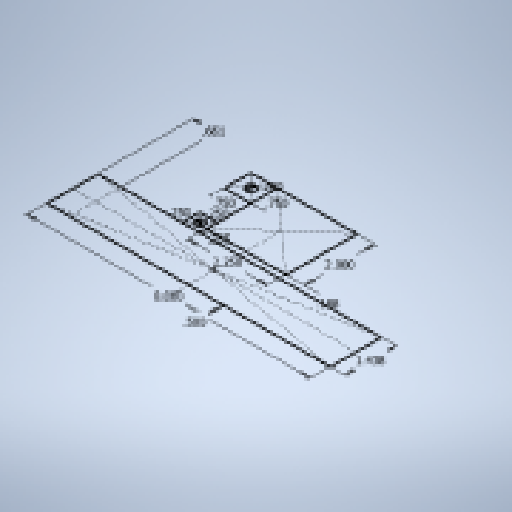
# Autodesk Inventor part: Chassis
Saved by Autodesk Inventor 2023.1 (Build 271208000, 208)
## iProperties
Created: 2022-12-23
Part Number: Chassis
Material: UHMW, White
Document SubType Name: Modeling
Designer: Nathan Cai
Density: 0.94 g/cm^3
Appearance: Smooth - White
Author: Nathan Cai
Autodesk Inventor part; units mm, degrees
ref_plane "YZ Plane" through (0, 0, 0) normal (1, 0, 0) x (0, 1, 0)
ref_plane "XZ Plane" through (0, 0, 0) normal (0, 1, 0) x (-1, 0, 0)
ref_plane "XY Plane" through (0, 0, 0) normal (0, 0, 1) x (1, 0, 0)
sketch "Sketch1" plane through (0, 0, 0) normal (0, 1, 0) x (-1, 0, 0)
  line L0 (28.575, -103.1875) -> (-28.575, -103.1875) construction
  line L1 (-28.575, -103.1875) -> (-28.575, -52.3875)
  line L2 (-28.575, -52.3875) -> (28.575, -52.3875)
  line L3 (28.575, -52.3875) -> (28.575, -103.1875)
  line L4 (28.575, -103.1875) -> (-28.575, -52.3875) construction
  line L5 (-28.575, -103.1875) -> (28.575, -52.3875) construction
  line L6 (0, -77.7875) -> (0, 0) construction
  line L7 (47.625, -103.1875) -> (28.575, -103.1875)
  line L8 (28.575, -103.1875) -> (28.575, -84.1375)
  line L9 (28.575, -84.1375) -> (47.625, -84.1375) construction
  line L10 (47.625, -84.1375) -> (47.625, -103.1875) construction
  line L11 (47.625, -103.1875) -> (28.575, -84.1375) construction
  line L12 (28.575, -103.1875) -> (47.625, -84.1375) construction
  circle A0 centre (38.1, -93.6625) radius 3.556
  line L13 (101.6, -49.2125) -> (-101.6, -49.2125)
  line L14 (-101.6, -49.2125) -> (-101.6, -12.7)
  line L15 (-101.6, -12.7) -> (101.6, -12.7)
  line L16 (101.6, -12.7) -> (101.6, -49.2125)
  line L17 (101.6, -49.2125) -> (-101.6, -12.7) construction
  line L18 (-101.6, -49.2125) -> (101.6, -12.7) construction
  line L19 (84.8, -49.2125) -> (84.8, -12.7) construction
  line L20 (-101.6, -30.9563) -> (101.6, -30.9563) construction
  circle A1 centre (34.925, -55.5625) radius 3.3655
  line L21 (41.275, -61.9125) -> (28.575, -61.9125)
  line L22 (28.575, -61.9125) -> (28.575, -49.2125)
  line L23 (28.575, -49.2125) -> (41.275, -49.2125)
  line L24 (41.275, -49.2125) -> (41.275, -61.9125)
  line L25 (41.275, -61.9125) -> (28.575, -49.2125) construction
  line L26 (28.575, -61.9125) -> (41.275, -49.2125) construction
  line L27 (34.925, -55.5625) -> (34.925, -7.9375) construction
  line L28 (41.275, -12.7) -> (28.575, -12.7)
  line L29 (28.575, -12.7) -> (28.575, -3.175) construction
  line L30 (28.575, -3.175) -> (41.275, -3.175)
  line L31 (41.275, -3.175) -> (41.275, -12.7)
  line L32 (41.275, -12.7) -> (28.575, -3.175) construction
  line L33 (28.575, -12.7) -> (41.275, -3.175) construction
  circle A2 centre (34.925, -7.9375) radius 3.3655
  circle A3 centre (38.1, -93.6625) radius 9.525
  line L34 (101.6, -49.2125) -> (60.325, -49.2125)
  line L35 (60.325, -49.2125) -> (60.325, -68.2625) construction
  line L36 (60.325, -68.2625) -> (101.6, -68.2625)
  line L37 (101.6, -68.2625) -> (101.6, -49.2125)
  line L38 (41.275, -52.3875) -> (60.325, -52.3875)
  line L39 (101.6, -7.9375) -> (41.275, -7.9375) construction
  line L40 (101.6, -7.9375) -> (101.6, -12.7)
  line L41 (101.6, -7.9375) -> (41.275, -3.175)
  line L42 (92.075, -49.2125) -> (92.075, -12.7)
  line L43 (60.325, -68.2625) -> (46.747, -97.6568)
  line L44 (34.925, -61.9125) -> (34.925, -84.6822)
  line L45 (57.166, -52.3875) -> (42.0943, -85.0155)
  line L46 (28.575, -3.175) -> (0, -3.175)
  circle A4 centre (60.325, -61.9125) radius 1.1906
  line L47 (101.6, -61.9125) -> (84.8, -61.9125)
  line L48 (84.8, -61.9125) -> (84.8, -36.5125)
  line L49 (84.8, -36.5125) -> (101.6, -36.5125)
  line L50 (101.6, -36.5125) -> (101.6, -61.9125)
  line L51 (84.8, -49.2125) -> (101.6, -49.2125) construction
  line L52 (84.8, -61.9125) -> (65.75, -61.9125)
  line L53 (65.75, -61.9125) -> (65.75, -36.5125)
  line L54 (65.75, -36.5125) -> (84.8, -36.5125)
  line L55 (84.8, -36.5125) -> (84.8, -61.9125)
  circle A5 centre (60.325, -36.5125) radius 1.1906
  line L56 (96.8375, -36.5125) -> (96.8375, -12.7) construction
  circle A6 centre (96.8375, -33.3375) radius 1.1906
  circle A7 centre (96.8375, -12.7) radius 1.1906
  circle A8 centre (60.325, -36.5125) radius 3.175
  line L57 (60.325, -33.3375) -> (92.075, -33.3375)
  line L58 (57.166, -36.1945) -> (57.166, -52.3875)
  line L59 (-47.625, -103.1875) -> (-28.575, -103.1875)
  circle A9 centre (-38.1, -93.6625) radius 3.556
  circle A10 centre (-34.925, -55.5625) radius 3.3655
  line L60 (-41.275, -61.9125) -> (-28.575, -61.9125)
  line L61 (-41.275, -49.2125) -> (-41.275, -61.9125)
  line L62 (-28.575, -3.175) -> (-41.275, -3.175)
  circle A11 centre (-34.925, -7.9375) radius 3.3655
  circle A12 centre (-38.1, -93.6625) radius 9.525
  line L63 (-60.325, -68.2625) -> (-101.6, -68.2625)
  line L64 (-101.6, -68.2625) -> (-101.6, -49.2125)
  line L65 (-41.275, -52.3875) -> (-60.325, -52.3875)
  line L66 (-101.6, -7.9375) -> (-41.275, -3.175)
  line L67 (-92.075, -49.2125) -> (-92.075, -12.7)
  line L68 (-60.325, -68.2625) -> (-46.747, -97.6568)
  line L69 (-34.925, -61.9125) -> (-34.925, -84.6822)
  line L70 (-57.166, -52.3875) -> (-42.0943, -85.0155)
  line L71 (-28.575, -3.175) -> (0, -3.175)
  circle A13 centre (-60.325, -61.9125) radius 1.1906
  line L72 (-101.6, -61.9125) -> (-84.8, -61.9125)
  line L73 (-84.8, -61.9125) -> (-84.8, -36.5125)
  line L74 (-84.8, -36.5125) -> (-101.6, -36.5125)
  line L75 (-84.8, -61.9125) -> (-65.75, -61.9125)
  line L76 (-65.75, -61.9125) -> (-65.75, -36.5125)
  line L77 (-65.75, -36.5125) -> (-84.8, -36.5125)
  circle A14 centre (-60.325, -36.5125) radius 1.1906
  circle A15 centre (-96.8375, -33.3375) radius 1.1906
  circle A16 centre (-96.8375, -12.7) radius 1.1906
  circle A17 centre (-60.325, -36.5125) radius 3.175
  line L78 (-60.325, -33.3375) -> (-92.075, -33.3375)
  line L79 (-57.166, -36.1945) -> (-57.166, -52.3875)
  line L80 (-101.6, -7.9375) -> (-101.6, -12.7)
  line L81 (41.275, -61.9125) -> (62.6618, -38.662)
  line L82 (-41.275, -61.9125) -> (-62.6618, -38.662)
  circle A18 centre (96.8375, -65.0875) radius 1.1906
  circle A19 centre (96.8375, -65.0875) radius 3.175 construction
  line L83 (87.975, -63.5) -> (84.8, -63.5)
  line L84 (84.8, -63.5) -> (84.8, -34.925)
  line L85 (84.8, -34.925) -> (87.975, -34.925)
  line L86 (87.975, -34.925) -> (87.975, -63.5)
  line L87 (87.975, -63.5) -> (84.8, -34.925) construction
  line L88 (84.8, -63.5) -> (87.975, -34.925) construction
  line L89 (-84.8, -61.9125) -> (-84.8, -36.5125)
  line L90 (-84.8, -36.5125) -> (-84.8, -61.9125)
  circle A20 centre (-96.8375, -65.0875) radius 1.1906
  circle A21 centre (-96.8375, -65.0875) radius 3.175
  line L91 (-87.975, -63.5) -> (-84.8, -63.5)
  line L92 (-84.8, -63.5) -> (-84.8, -34.925)
  line L93 (-84.8, -34.925) -> (-87.975, -34.925)
  line L94 (-87.975, -34.925) -> (-87.975, -63.5)
  line L95 (-87.975, -63.5) -> (-84.8, -34.925) construction
  line L96 (-84.8, -63.5) -> (-87.975, -34.925) construction
  point P0 (0, -30.9563)
  point P1 (-57.166, -49.2125)
  point P2 (-92.075, -12.7)
  point P3 (57.166, -49.2125)
  point P4 (38.1, -103.1875)
  point P5 (-38.1, -103.1875)
  point P6 (-50.0365, -52.3875)
  point P7 (50.0365, -52.3875)
  point P8 (86.3875, -49.2125)
  point P9 (-84.8, -49.2125)
  point P10 (-84.8, -49.2125)
  point P11 (-86.3875, -49.2125)
  dimension "d0" = 57.15
  dimension "d1" = 50.8
  dimension "d2" = 19.05
  dimension "d3" = 19.05
  dimension "d4" = 7.112
  dimension "d7" = 203.2
  dimension "d8" = 36.5125
  dimension "d9" = 3.175
  dimension "d10" = 16.8
  dimension "d11" = 6.731
  dimension "d12" = 6.35
  dimension "d13" = 6.35
  dimension "d14" = 12.7
  dimension "d15" = 12.7
  dimension "d16" = 9.525
  dimension "d17" = 6.731
  dimension "d18" = 41.275
  dimension "d19" = 19.05
  dimension "d20" = 3.175
  dimension "d21" = 9.525
  dimension "d23" = 9.525
  dimension "d24" = 2.3813
  dimension "d25" = 6.35
  dimension "d26" = 16.8
  dimension "d27" = 25.4
  dimension "d29" = 19.05
  dimension "d32" = 25.4
  dimension "d37" = 4.7625
  dimension "d38" = 2.3813
  dimension "d39" = 2.3813
  dimension "d40" = 6.35
  dimension "d41" = 3.175
  dimension "d51" = 6.35
  dimension "d52" = 3.175
  dimension "d53" = 28.575
  dimension "d54" = 6.35
  constraints: 194 end point, 52 symmetric about line, 31 point on line, 22 centre point, 20 parallel, 18 midpoint, 17 perpendicular, 11 point on circle, 9 horizontal, 7 coincident, 4 tangent, 3 vertical, 1 concentric, 14 other
  measures "d0" distance of L1.end L2.end
  measures "d1" distance of L0.end L1.end
  measures "d2" distance of L8.end L9.end
  measures "d3" distance of L7.end L8.end
  measures "d4" diameter of A0
  measures "d7" distance of L14.end L15.end
  measures "d8" distance of L13.end L14.end
  measures "d9" distance between parallel lines of L13 L2
  measures "d10" distance between parallel lines of L16 L19
  measures "d11" diameter of A1
  measures "d12" distance from line of L3 L27.start
  measures "d13" distance from line of L13 L27.start
  measures "d14" distance from line of L6.end L15
  measures "d15" distance of L29.end L30.end
  measures "d16" distance of L28.end L29.end
  measures "d17" diameter of A2
  measures "d18" distance of L36.end L35.end
  measures "d19" distance of L35.end L34.end
  measures "d20" distance between parallel lines of L13 L38
  measures "d21" distance between parallel lines of L16 L42
  measures "d23" distance between parallel lines of L43 L45
  measures "d24" diameter of A4
  measures "d25" distance from line of L36 A4.centre
  measures "d26" distance of L48.end L49.end
  measures "d27" distance of L47.end L48.end
  measures "d29" distance of L53.end L54.end
  measures "d32" distance of A4.centre A5.centre
  measures "d37" distance between parallel lines of L16 L56
  measures "d38" diameter of A6
  measures "d39" diameter of A7
  measures "d40" diameter of A8
  measures "d41" distance from line of L49 A6.centre
  measures "d51" diameter of A19
  measures "d52" distance of L84.end L85.end
  measures "d53" distance of L83.end L84.end
  measures "d54" distance between parallel lines of L36 L52
extrude "Extrusion1" add sketch "Sketch1" along normal blind 25.4 contours L59 A12 L1 | A12 L69 L60 L1 | A12 | L60 L61 L13 L22 L2 L1 | L68 L63 A21 L72 L94 L91 L92 L75 L76 L13 L79 L70 A12 | L22 L13 L24 L21 L3 | L82 L65 L61 | L79 L13 L82 L65 | L63 L64 L72 A21 | A21 | L21 L44 A3 L3 | L65 L82 L13 L61 | L13 L76 L77 L92 L93 L94 L74 L67 L78 A17 L82 L79 | L72 L64 L13 L94 | L13 L81 L38 L24 | L82 A17 L79 | A3 L7 L3 | A3 | L24 L38 L81 | L13 L58 L38 L81 | A17 L79 | L14 L74 L67 L13 | L13 L67 L74 L94 | L45 L58 L13 L53 L52 L84 L83 L86 L47 L37 L36 L43 A3 | L58 L81 A8 L57 L42 L49 L86 L85 L84 L54 L53 L13 | L58 A8 L81 | L14 L15 A16 L67 L74 | L58 A8 | L80 L66 L62 L71 L46 L30 L31 L15 A16 | L47 L86 L13 L37 | L86 L49 L42 L13 | L42 L15 A7 L16 L49 | L31 L41 L40 L15 A7 | L13 L42 L49 L16 | A4 | A13 picked at (-57.8908, -35.9532) picked at (62.7947, -36.8671)
fillet "Fillet1" radius 3.175 24 edges at (-42.0943, 12.7, -85.0155) (-34.925, 12.7, -84.6822) (-34.925, 12.7, -61.9125) (-41.275, 12.7, -61.9125) (-57.166, 12.7, -52.3875) (42.0943, 12.7, -85.0155) (34.925, 12.7, -84.6822) (34.925, 12.7, -61.9125) (41.275, 12.7, -61.9125) (57.166, 12.7, -52.3875) (-57.166, 12.7, -49.2125) (57.166, 12.7, -49.2125) (92.075, 12.7, -33.3375) (92.075, 12.7, -12.7) (-92.075, 12.7, -33.3375) (-92.075, 12.7, -12.7) (-101.6, 12.7, -7.9375) (101.6, 12.7, -7.9375) (41.275, 12.7, -3.175) (-41.275, 12.7, -3.175) (-50.0365, 12.7, -52.3875) (50.0365, 12.7, -52.3875) (-101.6, 12.7, -68.2625) (101.6, 12.7, -68.2625)
fillet "Fillet2" radius 6.35 4 edges at (-28.575, 12.7, -103.1875) (28.575, 12.7, -103.1875) (-28.575, 12.7, -52.3875) (28.575, 12.7, -52.3875)
fillet "Fillet3" radius 12.7 2 edges at (-60.325, 12.7, -68.2625) (60.325, 12.7, -68.2625)
sketch "Sketch2" plane through (-87.975, 0, -36.5125) normal (1, 0, 0) x (0, 0, -1)
  circle A0 centre (12.7, 12.7) radius 11
  line L0 (-1.5875, 25.4) -> (26.9875, 25.4) projected
  line L1 (-1.5875, 0) -> (26.9875, 0) projected
  line L2 (12.7, 25.4) -> (12.7, 0) construction
  line L3 (22.225, 22.225) -> (3.175, 22.225) construction
  line L4 (3.175, 22.225) -> (3.175, 3.175) construction
  line L5 (3.175, 3.175) -> (22.225, 3.175) construction
  line L6 (22.225, 3.175) -> (22.225, 22.225) construction
  line L7 (22.225, 22.225) -> (3.175, 3.175) construction
  line L8 (3.175, 22.225) -> (22.225, 3.175) construction
  circle A1 centre (22.225, 3.175) radius 1.7526
  circle A2 centre (3.175, 3.175) radius 1.7526
  circle A3 centre (22.225, 22.225) radius 1.7526
  circle A4 centre (3.175, 22.225) radius 1.7526
  point P0 (-36.5125, 0)
  dimension "d47" = 22
  dimension "d56" = 19.05
  dimension "d57" = 19.05
  dimension "d58" = 3.5052
  dimension "d61" = 19.05
  dimension "d64" = 19.05
  constraints: 14 end point, 5 centre point, 5 midpoint, 2 horizontal, 2 parallel, 1 coincident, 1 perpendicular, 1 vertical, 6 other
  measures "d47" diameter of A0
  measures "d56" distance of L5.end L4.end
  measures "d57" distance of L4.end L3.end
  measures "d58" diameter of A1
  measures "d61" distance of A1.centre A2.centre
  measures "d64" distance of A1.centre A3.centre
extrude "Extrusion2" cut sketch "Sketch2" against normal through all
fillet "Fillet4" radius 3.175 4 edges at (65.75, 12.7, -61.9125) (65.75, 12.7, -36.5125) (-65.75, 12.7, -36.5125) (-65.75, 12.7, -61.9125)
fillet "Fillet5" radius 1.5875 4 edges at (-84.8, 12.7, -61.9125) (-84.8, 12.7, -36.5125) (84.8, 12.7, -61.9125) (84.8, 12.7, -36.5125)
equation "\"d37\" = 0.5 * d21"
equation "\"d38\" = d24"
equation "\"d39\" = d24"
body "Solid1"
